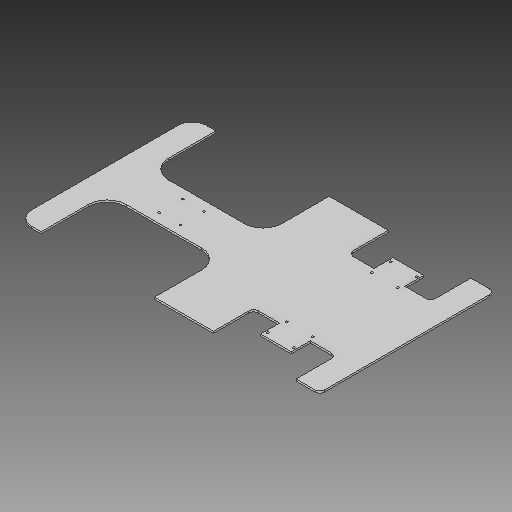
# Autodesk Inventor part: 00-01-Платформа
Saved by Autodesk Inventor 2018 (Build 220112000, 112)
## iProperties
Part Number: 00-01-Платформа
Material: Типовые
Document SubType Name: Modeling
Designer: sbnnl
Density: 1 g/cm^3
Appearance: По умолчанию
Author: sbnnl
Autodesk Inventor part; units mm, degrees
ref_plane "YZ Plane" through (0, 0, 0) normal (1, 0, 0) x (0, 1, 0)
ref_plane "XZ Plane" through (0, 0, 0) normal (0, 1, 0) x (-1, 0, 0)
ref_plane "XY Plane" through (0, 0, 0) normal (0, 0, 1) x (1, 0, 0)
sketch "Эскиз1" plane through (0, 0, 0) normal (0, 1, 0) x (-1, 0, 0)
  line L0 (0, 0) -> (62.2951, 0) construction
  line L1 (-40, 45) -> (-200, 45)
  line L2 (-200, -45) -> (-40, -45)
  circle A0 centre (-90, 25) radius 2.25
  line L3 (-90, 25) -> (-135, 25) construction
  circle A1 centre (-135, 25) radius 2.25
  circle A2 centre (-90, -25) radius 2.25
  circle A3 centre (-135, -25) radius 2.25
  line L4 (0, 185) -> (20, 185)
  line L5 (50, 155) -> (50, -155)
  line L6 (20, -185) -> (0, -185)
  line L7 (0, 85) -> (0, 185)
  arc A4 (50, 155) -> (20, 185) centre (20, 155) ccw
  arc A5 (20, -185) -> (50, -155) centre (20, -155) ccw
  line L8 (-240, 185) -> (-365, 185)
  line L9 (-590, 185) -> (-590, -185)
  line L10 (-590, -185) -> (-540, -185)
  line L11 (-240, 85) -> (-240, 185)
  arc A6 (-40, 45) -> (0, 85) centre (-40, 85) ccw
  line L12 (0, -185) -> (0, -85)
  arc A7 (0, -85) -> (-40, -45) centre (-40, -85) ccw
  arc A8 (-240, 85) -> (-200, 45) centre (-200, 85) ccw
  line L13 (-240, -185) -> (-240, -85)
  arc A9 (-200, -45) -> (-240, -85) centre (-200, -85) ccw
  line L14 (-365, 185) -> (-365, 100)
  line L15 (-365, 100) -> (-420, 100)
  line L16 (-420, 100) -> (-420, 140)
  line L17 (-420, 140) -> (-485, 140)
  line L18 (-485, 140) -> (-485, 100)
  line L19 (-485, 100) -> (-540, 100)
  line L20 (-540, 100) -> (-540, 185)
  line L21 (-495.3156, 130) -> (-414.5161, 130) construction
  circle A10 centre (-480, 130) radius 2.25
  circle A11 centre (-425, 130) radius 2.25
  line L22 (-452.5, 140) -> (-452.5, 103.3214) construction
  circle A12 centre (-480, 90) radius 2.25
  circle A13 centre (-425, 90) radius 2.25
  line L23 (-540, 185) -> (-590, 185)
  line L24 (-365, 185) -> (-540, 185) construction
  line L25 (-365, -185) -> (-365, -100)
  line L26 (-365, -100) -> (-420, -100)
  line L27 (-420, -100) -> (-420, -140)
  line L28 (-420, -140) -> (-485, -140)
  line L29 (-485, -140) -> (-485, -100)
  line L30 (-485, -100) -> (-540, -100)
  line L31 (-540, -100) -> (-540, -185)
  circle A14 centre (-480, -130) radius 2.25
  circle A15 centre (-425, -130) radius 2.25
  circle A16 centre (-480, -90) radius 2.25
  circle A17 centre (-425, -90) radius 2.25
  line L32 (-540, -185) -> (-365, -185) construction
  line L33 (-365, -185) -> (-240, -185)
  point P0 (50, 185)
  dimension "d10" = 4.5
  dimension "d11" = 45
  dimension "d12" = 25
  dimension "d13" = 90
  dimension "d14" = 50
  dimension "d15" = 370
  dimension "d16" = 30
  dimension "d20" = 350
  dimension "d21" = 40
  dimension "d22" = 40
  dimension "d23" = 90
  dimension "d24" = 40
  dimension "d25" = 40
  dimension "d26" = 240
  dimension "d27" = 50
  dimension "d28" = 55
  dimension "d29" = 45
  dimension "d30" = 65
  dimension "d31" = 55
  dimension "d32" = 85
  dimension "d33" = 4.5
  dimension "d34" = 55
  dimension "d35" = 10
  dimension "d38" = 40
  constraints: 68 end point, 18 centre point, 15 symmetric about line, 13 parallel, 12 point on circle, 12 tangent, 11 perpendicular, 11 point on line, 8 horizontal, 6 collinear, 5 vertical, 3 equal radius, 1 coincident, 1 midpoint, 12 other
  measures "d10" diameter of A1
  measures "d11" distance of L3.start L3.end
  measures "d12" distance between parallel lines of L0 L3
  measures "d13" horizontal distance of L3.start L0.start
  measures "d14" distance of L4.start point (50, 185)
  measures "d15" distance between parallel lines of L6 L4
  measures "d16" radius of A4
  measures "d20" distance of L8.start L9.start
  measures "d21" radius of A6
  measures "d22" radius of A7
  measures "d23" distance between parallel lines of L2 L1
  measures "d24" radius of A8
  measures "d25" radius of A9
  measures "d26" distance between parallel lines of L11 L7
  measures "d27" distance between parallel lines of L9 L20
  measures "d28" distance between parallel lines of L18 L20
  measures "d29" distance between parallel lines of L17 L8
  measures "d30" distance between parallel lines of L16 L18
  measures "d31" distance between parallel lines of L14 L16
  measures "d32" distance between parallel lines of L19 L8
  measures "d33" diameter of A10
  measures "d34" distance of A11.centre A10.centre
  measures "d35" distance between parallel lines of L21 L17
  measures "d38" distance of A10.centre A12.centre
extrude "Выдавливание3" add sketch "Эскиз1" along normal blind 4
fillet "Сопряжение1" radius 10 4 edges at (365, 2, 100) (540, 2, 100) (540, 2, -100) (365, 2, -100)
fillet "Сопряжение2" radius 10 2 edges at (590, 2, -185) (590, 2, 185)
equation "\"d22\" = d21"
equation "\"d24\" = d21"
equation "\"d25\" = d21"
